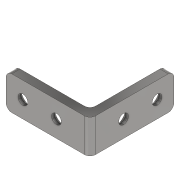
# Autodesk Inventor part: Bracket
Saved by Autodesk Inventor 2020 (Build 240168000, 168)
## iProperties
Created: 2020-10-10
Part Number: Bracket
Material: Generic
Document SubType Name: Modeling
Designer: ferrerx
Density: 1 g/cm^3
Appearance: Steel - Polished
Author: ferrerx
Autodesk Inventor part; units mm, degrees
ref_plane "YZ Plane" through (0, 0, 0) normal (1, 0, 0) x (0, 1, 0)
ref_plane "XZ Plane" through (0, 0, 0) normal (0, 1, 0) x (-1, 0, 0)
ref_plane "XY Plane" through (0, 0, 0) normal (0, 0, 1) x (1, 0, 0)
sketch "Sketch1" plane through (0, 0, 0) normal (0, 1, 0) x (-1, 0, 0)
  line L0 (0, 0) -> (30, 0)
  line L1 (30, 0) -> (30, -3)
  line L2 (30, -3) -> (3, -3)
  line L3 (3, -3) -> (3, -30)
  line L4 (3, -30) -> (0, -30)
  line L5 (0, -30) -> (0, 0)
  dimension "d0" = 3
  dimension "d1" = 3
  dimension "d4" = 30
  dimension "d5" = 30
  constraints: 12 end point, 5 perpendicular, 1 horizontal
  measures "d0" distance between parallel lines of L0 L2
  measures "d1" distance between parallel lines of L5 L3
  measures "d4" distance of L0.start L0.end
  measures "d5" distance of L4.end L0.start
extrude "Extrusion1" add sketch "Sketch1" along normal blind 12
sketch "Sketch2" plane through (-3, 0, -30) normal (-1, 0, 0) x (0, 0, 1)
  line L0 (0, 0) -> (0, 12) projected
  line L1 (0, 6) -> (27, 6) construction
  line L2 (27, 0) -> (27, 12) projected
  circle A0 centre (6, 6) radius 1.75
  circle A1 centre (18, 6) radius 1.75
  point P0 (30, 0)
  dimension "d8" = 3.5
  dimension "d9" = 3.5
  dimension "d10" = 6
  dimension "d11" = 12
  constraints: 2 centre point, 2 end point, 2 midpoint, 2 point on line
  measures "d8" diameter of A0
  measures "d9" diameter of A1
  measures "d10" distance from line of L0 A0.centre
  measures "d11" distance of A1.centre A0.centre
extrude "Extrusion2" cut sketch "Sketch2" against normal blind 12
sketch "Sketch3" plane through (-3, 0, -3) normal (0, 0, -1) x (-1, 0, 0)
  line L0 (27, 0) -> (27, 12) projected
  line L1 (27, 6) -> (0, 6) construction
  line L2 (0, 0) -> (0, 12) projected
  circle A0 centre (21, 6) radius 1.75
  circle A1 centre (9, 6) radius 1.75
  point P0 (-3, 0)
  dimension "d14" = 6
  dimension "d15" = 12
  dimension "d16" = 3.5
  dimension "d17" = 3.5
  constraints: 2 centre point, 2 end point, 2 midpoint, 2 point on line
  measures "d14" distance from line of L0 A0.centre
  measures "d15" distance of A0.centre A1.centre
  measures "d16" diameter of A0
  measures "d17" diameter of A1
extrude "Extrusion3" cut sketch "Sketch3" against normal blind 12
chamfer "Chamfer1" distance 2 angle 45 4 edges at (-22.25, 6, -3) (-10.25, 6, -3) (-3, 6, -13.75) (-3, 6, -25.75)
fillet "Fillet1" radius 2 6 edges at (-1.5, 12, -30) (-1.5, 0, -30) (-30, 12, -1.5) (-30, 0, -1.5) (-3, 6, -3) (0, 6, 0)
body "Solid1"
